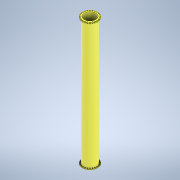
# Autodesk Inventor part: diam1m_len10m_xcirc_bolts_temp
Saved by Autodesk Inventor 2022 (Build 260153000, 153)
## iProperties
Created: 2021-12-16
Part Number: diam1m_len10m_xcirc_bolts_temp
Material: Steel
Document SubType Name: Modeling
Designer: jpc
Density: 7.85 g/cm^3
Appearance: Smooth - Yellow
Mass: 5.38964e+06 g
Surface Area: 633977 cm^2
Volume: 686578 cm^3
Author: jpc
Autodesk Inventor part; units mm, degrees
ref_plane "YZ Plane" through (0, 0, 0) normal (1, 0, 0) x (0, 1, 0)
ref_plane "XZ Plane" through (0, 0, 0) normal (0, 1, 0) x (-1, 0, 0)
ref_plane "XY Plane" through (0, 0, 0) normal (0, 0, 1) x (1, 0, 0)
sketch "Sketch7" plane through (0, 0, 0) normal (0, 1, 0) x (-1, 0, 0)
  circle A0 centre (0, 0) radius 500
  circle A1 centre (0, 0) radius 450
  dimension "diamO" = 1000
  dimension "diamI" = 900
  constraints: 2 centre point, 2 coincident
  measures "diamO" diameter of A0
  measures "diamI" diameter of A1
extrude "Cylinder" add sketch "Sketch7" along normal blind 10000
sketch "Sketch8" plane through (0, 0, 0) normal (0, -1, 0) x (1, 0, 0)
  circle A0 centre (0, 0) radius 450 projected
  circle A1 centre (0, 0) radius 600
  dimension "d38" = 1200
  constraints: 1 centre point, 1 coincident
  measures "d38" diameter of A1
extrude "Endcap" add sketch "Sketch8" against normal blind 50
chamfer "EndcapChamfer" distance 10 angle 45 1 edges at (-600, 0, 0)
sketch "Sketch9" plane through (0, 50, 0) normal (0, 1, 0) x (1, 0, 0)
  circle A0 centre (0, 0) radius 600 construction
  circle A1 centre (0, 0) radius 450 construction
  circle A2 centre (0, 0) radius 500 construction
  circle A3 centre (0, 0) radius 600 construction
  line L0 (0, 600) -> (0, 500) construction
  circle A4 centre (0, 0) radius 500 construction
  circle A5 centre (0, 550) radius 25
  dimension "d44" = 1200
  dimension "d45" = 1000
  dimension "d46" = 50
  constraints: 2 end point, 2 vertical alignment, 1 centre point, 1 line through centre, 1 midpoint, 1 vertical, 2 other
  measures "d44" diameter of A0
  measures "d45" diameter of A2
  measures "d46" diameter of A5
extrude "BoltHole" cut sketch "Sketch9" against normal through all
pattern_circular "BoltHoles" count 24 over 360 about axis through (0, -10, 0) along (0, 1, 0) of "BoltHole"
ref_plane "Midplane" through (0, 5000, 0) normal (0, -1, 0) x (1, 0, 0)
mirror "MirroredEndcap" about plane through (0, 5000, 0) normal (0, -1, 0) of "Endcap", "EndcapChamfer", "BoltHole", "BoltHoles"
sketch "Sketch10" plane through (0, 50, 0) normal (0, 1, 0) x (1, 0, 0)
  circle A0 centre (0, 550) radius 25 construction
  circle A1 centre (0, 550) radius 31.25 construction
  line L0 (-31.25, 568.0422) -> (0, 586.0844)
  line L1 (0, 586.0844) -> (31.25, 568.0422)
  line L2 (31.25, 568.0422) -> (31.25, 531.9578)
  line L3 (31.25, 531.9578) -> (0, 513.9156)
  line L4 (0, 513.9156) -> (-31.25, 531.9578)
  line L5 (-31.25, 531.9578) -> (-31.25, 568.0422)
  point P0 (0, 0)
  point P1 (-31.25, 550)
  dimension "d53" = 62.5
  dimension "d52" = 50
  constraints: 12 end point, 2 coincident, 1 horizontal alignment, 1 midpoint, 1 vertical, 15 other
  measures "d52" diameter of A0
extrude "BoltHead" add sketch "Sketch10" along normal blind 37.5 separate body
sketch "Sketch11" plane through (0, 50, 0) normal (0, -1, 0) x (1, 0, 0)
  circle A0 centre (0, -550) radius 25 projected
  point P0 (0, 0)
extrude "BoltThread" add sketch "Sketch11" along normal blind 175 bodies 2
ref_plane "JoinedEndcapPlane" through (0, -50, 0) normal (0, -1, 0) x (1, 0, 0)
sketch "Sketch12" plane through (0, -50, 0) normal (0, -1, 0) x (1, 0, 0)
  line L0 (-31.25, -531.9578) -> (0, -513.9156) projected
  line L1 (-31.25, -568.0422) -> (-31.25, -531.9578) projected
  line L2 (0, -586.0844) -> (-31.25, -568.0422) projected
  line L3 (31.25, -568.0422) -> (0, -586.0844) projected
  line L4 (31.25, -531.9578) -> (31.25, -568.0422) projected
  line L5 (0, -513.9156) -> (31.25, -531.9578) projected
  point P0 (0, 0)
extrude "BoltNut" add sketch "Sketch12" along normal blind 37.5 bodies 2
chamfer "BoltThreadChamfer" distance 10 angle 45 1 edges at (-25, -125, -550)
pattern_circular "Circular Pattern5" count 24 over 360 about axis through (0, -10, 0) along (0, 1, 0) bodies 2
mirror "ReflectedBolts" about plane through (0, 5000, 0) normal (0, -1, 0) bodies 2 separate body
mirror "FixedBolts" about plane through (0, 10000, 0) normal (0, 1, 0) remove original yes bodies 3
sketch "Sketch13" plane through (0, 0, 0) normal (1, 0, 0) x (0, 1, 0)
  line L0 (10000, 600) -> (0, 600)
  line L1 (0, 600) -> (0, -600)
  line L2 (0, -600) -> (10000, -600)
  line L3 (10000, -600) -> (10000, 600)
  line L4 (50, -600) -> (50, 600) projected
  line L5 (10, 600) -> (10, -600) projected
  line L6 (10, 600) -> (10, -600) projected
  line L7 (0, -590) -> (0, 590) projected
  line L8 (10, 600) -> (50, 600) projected
  line L9 (-10000, 10600) -> (20000, 10600)
  line L10 (20000, 10600) -> (20000, -10600)
  line L11 (20000, -10600) -> (-10000, -10600)
  line L12 (-10000, -10600) -> (-10000, 10600)
  point P0 (0, 0)
  dimension "d67" = 1200
  dimension "d68" = 10000
  dimension "d69" = 10000
  constraints: 16 end point, 4 parallel, 2 collinear, 2 perpendicular, 1 horizontal, 3 other
  measures "d67" distance of L0.end L1.end
  measures "d68" distance of L0.start L0.end
  measures "d69" distance between parallel lines of L0 L9
extrude "TrimBolts" cut sketch "Sketch13" along normal through all both and the other way through all bodies 1 2 3
equation "\"d38\" = 1.2 * diamO"
equation "\"endcapThick\" = 0.005 * len"
equation "\"d41\" = -0.1 * diamI + 0.1 * diamO"
equation "\"d46\" = -0.25 * d45 + 0.25 * d44"
equation "\"d53\" = 1.25 * d52"
equation "\"boltThick\" = 0.75 * endcapThick"
equation "\"d56\" = 2 * endcapThick + 2 * boltThick"
equation "\"d59\" = boltThick"
equation "\"d61\" = -0.1 * diamI + 0.1 * diamO"
equation "\"d67\" = 1.2 * diamO"
equation "\"d68\" = len"
equation "\"d69\" = len"
equation "\"len\" = 10000"
